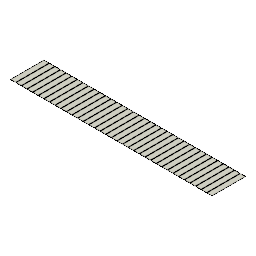
open keyboard v1 (Autodesk Fusion 360 design; units mm, degrees)
Autodesk Fusion 360 part; units mm, degrees
sketch "Sketch1" plane through (0, 0, 0) normal (0, 0, 1) x (1, 0, 0) in component "keys_white"
  line L0 (0, 0) -> (21.97, 0) construction
  line L1 (21.97, 0) -> (21.97, 132) construction
  line L2 (21.97, 132) -> (0, 132) construction
  line L3 (0, 132) -> (0, 0) construction
  line L4 (0.75, 132) -> (21.22, 132)
  line L5 (21.22, 132) -> (21.22, 0)
  line L6 (21.22, 0) -> (0.75, 0)
  line L7 (0.75, 0) -> (0.75, 132)
  dimension "d11" = 21.97
  dimension "d12" = 132
  dimension "d15" = 0.75
  dimension "d16" = 0.75
  constraint horizontal L0
  constraint vertical L1
  constraint horizontal L2
  constraint vertical L3
  constraint coincident L0.start L3.end
  constraint horizontal L4
  constraint vertical L5
  constraint horizontal L6
  constraint vertical L7
  constraint coincident L0 L5.end
  constraint coincident L2 L4.start
  measures "d11" distance of L0.start L0.end
  measures "d12" distance of L0.start L2.end
  measures "d15" distance of L3 L7
  measures "d16" distance of L1 L5
extrude "Extrude1" add sketch "Sketch1" along normal blind 0.6 makes body 1 in component "keys_white"
pattern_linear "R-Pattern1" count 36 spacing 21.97 along (1, 0, 0) of bodies 1 makes body 2 at (29.5433, 88, 0) makes body 3 at (51.5133, 88, 0) makes body 4 at (73.4833, 88, 0) makes body 5 at (95.4533, 88, 0) makes body 6 at (117.4233, 88, 0) makes body 7 at (139.3933, 88, 0) makes body 8 at (161.3633, 88, 0) makes body 9 at (183.3333, 88, 0) makes body 10 at (205.3033, 88, 0) makes body 11 at (227.2733, 88, 0) makes body 12 at (249.2433, 88, 0) makes body 13 at (271.2133, 88, 0) makes body 14 at (293.1833, 88, 0) makes body 15 at (315.1533, 88, 0) makes body 16 at (337.1233, 88, 0) makes body 17 at (359.0933, 88, 0) makes body 18 at (381.0633, 88, 0) makes body 19 at (403.0333, 88, 0) makes body 20 at (425.0033, 88, 0) makes body 21 at (446.9733, 88, 0) makes body 22 at (468.9433, 88, 0) makes body 23 at (490.9133, 88, 0) makes body 24 at (512.8833, 88, 0) makes body 25 at (534.8533, 88, 0) makes body 26 at (556.8233, 88, 0) makes body 27 at (578.7933, 88, 0) makes body 28 at (600.7633, 88, 0) makes body 29 at (622.7333, 88, 0) makes body 30 at (644.7033, 88, 0) makes body 31 at (666.6733, 88, 0) makes body 32 at (688.6433, 88, 0) makes body 33 at (710.6133, 88, 0) makes body 34 at (732.5833, 88, 0) makes body 35 at (754.5533, 88, 0) makes body 36 at (776.5233, 88, 0) in component "keys_white"
component "manual" placed x (1, 0, 0) y (0, 1, 0) z (0, 0, 1) at (0, 0, 0)
component "keys_white" placed x (1, 0, 0) y (0, 1, 0) z (0, 0, 1) at (0, 0, 0) in component "manual"
equation "n_keys = 61" comment "number of keys to generate"
equation "tot_key_width_black = ( 840 / 61 ) * 1 mm"
equation "tot_key_width_white = 23.47 mm"
equation "space = 1.5 mm"
equation "key_width_black = tot_key_width_black - space" comment "actual width of the black keys"
equation "key_width_white = tot_key_width_white - space" comment "actual width of the white keys"
equation "key_length_white = 50 mm" comment "length white keys extend beyond black"
equation "key_length_black = 82 mm - space" comment "length of black keys"
equation "key_length = key_length_black + key_length_white + space" comment "total length of white keys and manual"
equation "total_width = tot_key_width_black * n_keys"
equation "d11 = key_width_white"
equation "d12 = key_length"
equation "n_keys_white = n_keys - ( floor(n_keys / 12) * 5 )"
equation "n_keys_black = floor(n_keys / 12) * 5"
equation "d15 = space / 2"
equation "d16 = d15"
equation "d19 = n_keys_white"
equation "d21 = key_width_white"
